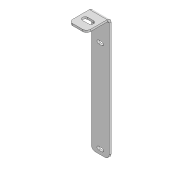
# Autodesk Inventor part: BREEZE-M30
Saved by Autodesk Inventor 2020 (Build 240168000, 168)
## iProperties
Created: 2020-04-15
Part Number: BREEZE-M30
Material: Generic
Document SubType Name: Sheet Metal
Designer: John K
Density: 1 g/cm^3
Sheet Metal Rule: Default_mm
Appearance: Default
Description: PCB BRACKET
Flat Pattern Width: 1.8 cm
Flat Pattern Length: 14.6524 cm
Flat Pattern Area: 26.3743 cm^2
Sheet Metal Width: 18.000 mm
Sheet Metal Length: 146.524 mm
Sheet Metal Area: 2637.430 mm^2
Author: John K
Autodesk Inventor part; units mm, degrees
ref_plane "YZ Plane" through (0, 0, 0) normal (1, 0, 0) x (0, 1, 0)
ref_plane "XZ Plane" through (0, 0, 0) normal (0, 1, 0) x (-1, 0, 0)
ref_plane "XY Plane" through (0, 0, 0) normal (0, 0, 1) x (1, 0, 0)
sketch "Sketch1" plane through (0, 0, 0) normal (0, 0, 1) x (1, 0, 0)
  line L0 (-9, -62.5) -> (9, -62.5)
  line L1 (9, -62.5) -> (9, 62.5)
  line L2 (9, 62.5) -> (-9, 62.5)
  line L3 (-9, 62.5) -> (-9, -62.5)
  line L4 (-9, -62.5) -> (9, 62.5) construction
  line L5 (9, -62.5) -> (-9, 62.5) construction
  point P0 (0, 0)
  dimension "d0" = 18
  dimension "d1" = 125
  measures "d0" distance of L2.end L1.end
  measures "d1" distance of L1.end L0.end
extrude "Plate1" add sketch "Sketch1" along normal blind 2
sketch "Sketch2" plane through (-9, 60.5, 0) normal (0, 1, 0) x (-1, 0, 0)
  line L0 (-18, 0) -> (0, 0)
  line L1 (0, 0) -> (0, 25)
  line L2 (0, 25) -> (-18, 25)
  line L3 (-18, 25) -> (-18, 0)
  constraints: 6 end point, 1 horizontal, 1 perpendicular, 1 vertical
edge flange "Flange1" height 25 angle 90 thickness 2 bend radius 2 thickness toward (0, 1, 0) relief tear relief width 2 relief depth 1 edges at (0, 62.5, 2) wall of the first edge with corners at (9, 60.5, 0) (-9, 60.5, 0) (-9, 60.5, 25) (9, 60.5, 25)
bend "Bend1"
corner "Corner1"
sketch "Sketch3" plane through (0, 0, 2) normal (0, 0, 1) x (1, 0, 0)
  line L0 (-1.75, -57.5) -> (1.75, -57.5) construction
  line L1 (-1.75, -59.2) -> (1.75, -59.2)
  line L2 (1.75, -55.8) -> (-1.75, -55.8)
  arc A0 (-1.75, -55.8) -> (-1.75, -59.2) centre (-1.75, -57.5) ccw
  arc A1 (1.75, -59.2) -> (1.75, -55.8) centre (1.75, -57.5) ccw
  line L3 (-1.75, 36.5) -> (1.75, 36.5) construction
  line L4 (-9, -62.5) -> (-9, 58.5) projected
  line L5 (-1.75, 34.8) -> (1.75, 34.8)
  line L6 (1.75, 38.2) -> (-1.75, 38.2)
  arc A2 (-1.75, 38.2) -> (-1.75, 34.8) centre (-1.75, 36.5) ccw
  arc A3 (1.75, 34.8) -> (1.75, 38.2) centre (1.75, 36.5) ccw
  line L7 (9, -62.5) -> (-9, -62.5) projected
  point P0 (0, 0)
  point P1 (0, -57.5)
  point P2 (0, 36.5)
  dimension "d13" = 94
  dimension "d14" = 5
  dimension "d15" = 3.4
  dimension "d16" = 3.5
  constraints: 16 end point, 8 point on circle, 8 tangent, 4 centre point, 3 parallel, 2 midpoint, 2 vertical alignment, 1 equal radius, 1 horizontal, 1 perpendicular
  measures "d13" distance between parallel lines of L0 L3
  measures "d14" distance between parallel lines of L7 L0
  measures "d15" diameter of A3
  measures "d16" distance of L0.start L0.end
extrude "Cut1" cut sketch "Sketch3" against normal blind 2
sketch "Sketch4" plane through (-9, 62.5, 25) normal (0, 1, 0) x (1, 0, 0)
  line L0 (12, 10.5) -> (6, 10.5) construction
  line L1 (12, 13.25) -> (6, 13.25)
  line L2 (6, 7.75) -> (12, 7.75)
  arc A0 (12, 7.75) -> (12, 13.25) centre (12, 10.5) ccw
  arc A1 (6, 13.25) -> (6, 7.75) centre (6, 10.5) ccw
  line L3 (18, 21) -> (18, 0) projected
  point P0 (9, 25)
  point P1 (9, 10.5)
  point P2 (18, 10.5)
  dimension "d19" = 5.5
  dimension "d20" = 6
  constraints: 8 end point, 4 point on circle, 4 tangent, 2 centre point, 2 midpoint, 1 horizontal, 1 horizontal alignment, 1 parallel, 1 vertical alignment
  measures "d19" diameter of A1
  measures "d20" distance of L0.start L0.end
extrude "Cut2" cut sketch "Sketch4" against normal blind 2
fillet "Fillet1" radius 4 4 edges at (-9, 61.5, 25) (9, 61.5, 25) (-9, -62.5, 1) (9, -62.5, 1)
equation "\"d17\" = Thickness"
equation "\"d21\" = Thickness"
equation "\"d2\" = Thickness"
equation "\"d3\" = BendReliefWidth"
equation "\"d4\" = BendReliefDepth"
equation "\"d5\" = MinimumRemnant"
equation "\"d6\" = TransitionRadius"
equation "\"d9\" = BendRadius"
equation "\"d10\" = CornerReliefSize"
equation "\"d11\" = GapSize"
equation "\"d12\" = JacobiRadiusSize"
equation "\"BendRadius\" = Thickness"
equation "\"BendReliefWidth\" = Thickness"
equation "\"BendReliefDepth\" = 0.5 * Thickness"
equation "\"CornerReliefSize\" = 4 * Thickness"
equation "\"MinimumRemnant\" = 2 * Thickness"
equation "\"TransitionRadius\" = BendRadius"
equation "\"JacobiRadiusSize\" = BendRadius"
equation "\"GapSize\" = Thickness"
equation "\"Thickness\" = 2"
body "Solid1"
